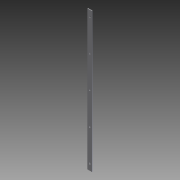
# Autodesk Inventor part: top panel
Saved by Autodesk Inventor 2012 (Build 160160000, 160)
## iProperties
Created: 2012-05-13
Part Number: top panel
Material: Default
Document SubType Name: Modeling
Designer: Puzzles
Density: 1 g/cm^3
Author: Puzzles
Autodesk Inventor part; units mm, degrees
ref_plane "YZ Plane" through (0, 0, 0) normal (1, 0, 0) x (0, 1, 0)
ref_plane "XZ Plane" through (0, 0, 0) normal (0, 1, 0) x (-1, 0, 0)
ref_plane "XY Plane" through (0, 0, 0) normal (0, 0, 1) x (1, 0, 0)
sketch "Sketch1" plane through (0, 0, 0) normal (0, 0, 1) x (1, 0, 0)
  line L0 (-9.525, 292.1) -> (9.525, 292.1)
  line L1 (9.525, 292.1) -> (9.525, -292.1)
  line L2 (9.525, -292.1) -> (-9.525, -292.1)
  line L3 (-9.525, -292.1) -> (-9.525, 292.1)
  point P0 (0, 0)
  point P1 (9.525, 0)
  point P2 (0, 292.1)
  dimension "d0" = 19.05
  dimension "d1" = 584.2
  constraints: 8 end point, 2 midpoint, 2 parallel, 1 horizontal, 1 horizontal alignment, 1 perpendicular, 1 vertical alignment
  measures "d0" distance of L0.start L0.end
  measures "d1" distance of L2.end L0.start
extrude "Extrusion1" add sketch "Sketch1" along normal blind 3
sketch "Sketch2" plane through (0, 0, 3) normal (0, 0, 1) x (1, 0, 0)
  line L0 (-9.525, 292.1) -> (9.525, 292.1) projected
  line L1 (9.525, -292.1) -> (-9.525, -292.1) projected
  point P0 (0, 0)
  point P1 (0, 266.7)
  point P2 (0, 133.35)
  point P3 (0, 0)
  point P4 (0, -133.35)
  point P5 (0, -266.7)
  dimension "d4" = 25.4
  dimension "d5" = 133.35
  dimension "d6" = 133.35
  dimension "d7" = 133.35
  dimension "d8" = 133.35
  dimension "d9" = 25.4
  measures "d4" distance from line of L0 point (0, 266.7)
  measures "d5" distance of point (0, 133.35) point (0, 266.7)
  measures "d6" distance of point (0, 133.35) point (0, 0)
  measures "d7" distance of point (0, -133.35) point (0, 0)
  measures "d8" distance of point (0, -266.7) point (0, -133.35)
  measures "d9" distance from line of L1 point (0, -266.7)
hole "Hole1" at (0, 266.7, 3) at (0, 133.35, 3) at (0, 0, 3) at (0, -133.35, 3) at (0, -266.7, 3) direction (0, 0, -1) diameter 6.35 end through all
body "Solid1"
